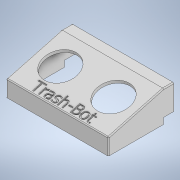
# Autodesk Inventor part: Ultrasonic_Sensor_Holder
Saved by Autodesk Inventor 2020 (Build 240168000, 168)
## iProperties
Created: 2023-02-02
Part Number: Ultrasonic_Sensor_Holder
Material: Generic
Document SubType Name: Modeling
Designer: Matthew Ng
Density: 1 g/cm^3
Appearance: Default
Author: Matthew Ng
Autodesk Inventor part; units mm, degrees
ref_plane "YZ Plane" through (0, 0, 0) normal (1, 0, 0) x (0, 1, 0)
ref_plane "XZ Plane" through (0, 0, 0) normal (0, 1, 0) x (-1, 0, 0)
ref_plane "XY Plane" through (0, 0, 0) normal (0, 0, 1) x (1, 0, 0)
sketch "Sketch1" plane through (0, 0, 0) normal (1, 0, 0) x (0, 1, 0)
  line L0 (0, 0) -> (8, 0)
  line L1 (15.2346, -27) -> (8, 0)
  line L2 (15.2346, -27) -> (15.2346, -32)
  line L3 (15.2346, -32) -> (0, -32)
  line L4 (0, -32) -> (0, 0)
  dimension "d8" = 8
  dimension "d26" = 5
  dimension "d27" = 32
  dimension "d28" = 15.2346
  dimension "d29" = 75
  constraints: 10 end point, 1 horizontal, 1 vertical
  measures "d8" distance of L0.start L0.end
  measures "d26" distance of L2.start L2.end
  measures "d27" distance of L3.end L0.start
  measures "d28" distance of L2.end L3.end
  measures "d29" angle of L3 L1
extrude "Extrusion1" add sketch "Sketch1" against normal blind 50
shell "Shell2" thickness 1.5 removed faces 2 at (-33.3333, 0, -10.6667) at (-33.3333, 5.0782, -32)
sketch "Sketch6" plane through (-50, 15.2346, -27) normal (0, 0.9659258, 0.258819) x (1, 0, 0)
  line L0 (25, -27.9525) -> (25, 4.8296) construction
  point P0 (50, -30.023)
  point P1 (12, -12.9525)
  point P2 (38, -12.9525)
  point P3 (12, -12.9525)
  dimension "d31" = 25.9999
  constraints: 2 end point, 1 coincident, 1 symmetric about line
  measures "d31" distance of point (38, -12.952) point (12, -12.952)
hole "Hole2" at (-38, 11.8823, -14.4889) at (-12, 11.8823, -14.4889) direction (0, -0.9659258, -0.258819) diameter 16 end through all
sketch "Sketch7" plane through (-50, 15.2346, -27) normal (0, 0.9659258, 0.258819) x (1, 0, 0)
  line L0 (12.3611, -21.6967) -> (37.6389, -21.6967) construction
  line L1 (37.6389, -21.6967) -> (37.6389, -26.9518) construction
  line L2 (37.6389, -26.9518) -> (12.3611, -26.9518) construction
  line L3 (12.3611, -26.9518) -> (12.3611, -21.6967) construction
  line L4 (11.8801, -26.9196) -> (11.8801, -22.5111)
  line L5 (11.8801, -22.5111) -> (10.2026, -22.5111)
  line L6 (10.2026, -22.5111) -> (10.2026, -21.9196)
  line L7 (10.2026, -21.9196) -> (14.222, -21.9196)
  line L8 (14.222, -21.9196) -> (14.222, -22.5111)
  line L9 (14.222, -22.5111) -> (12.5446, -22.5111)
  line L10 (12.5446, -22.5111) -> (12.5446, -26.9196)
  line L11 (12.5446, -26.9196) -> (11.8801, -26.9196)
  line L12 (16.6694, -23.8442) -> (16.637, -23.8442)
  spline S0 degree 2 poles (16.637, -23.8442) (16.564, -23.8239) (16.406, -23.8158) (16.2966, -23.8158) knots 0 0 0 1 2 2 2
  spline S1 degree 2 poles (16.2966, -23.8158) (16.0413, -23.8158) (15.5389, -24.0387) (15.312, -24.2575) knots 0 0 0 1 2 2 2
  line L13 (15.312, -24.2575) -> (15.312, -26.9196)
  line L14 (15.312, -26.9196) -> (14.6799, -26.9196)
  line L15 (14.6799, -26.9196) -> (14.6799, -23.1675)
  line L16 (14.6799, -23.1675) -> (15.312, -23.1675)
  line L17 (15.312, -23.1675) -> (15.312, -23.7267)
  spline S2 degree 2 poles (15.312, -23.7267) (15.6564, -23.4188) (16.171, -23.1675) (16.4141, -23.1675) knots 0 0 0 1 2 2 2
  spline S3 degree 2 poles (16.4141, -23.1675) (16.5113, -23.1675) (16.6086, -23.1756) (16.6694, -23.1878) knots 0 0 0 1 2 2 2
  line L18 (16.6694, -23.1878) -> (16.6694, -23.8442)
  spline S4 degree 2 poles (19.2504, -26.5225) (19.1734, -26.5792) (18.9141, -26.7818) (18.7925, -26.8426) knots 0 0 0 1 2 2 2
  spline S5 degree 2 poles (18.7925, -26.8426) (18.6264, -26.9317) (18.3144, -27.0249) (18.0308, -27.0249) knots 0 0 0 1 2 2 2
  spline S6 degree 2 poles (18.0308, -27.0249) (17.7998, -27.0249) (17.3825, -26.8507) (17.2245, -26.6927) knots 0 0 0 1 2 2 2
  spline S7 degree 2 poles (17.2245, -26.6927) (17.0746, -26.5387) (16.8922, -26.0849) (16.8922, -25.8337) knots 0 0 0 1 2 2 2
  spline S8 degree 2 poles (16.8922, -25.8337) (16.8922, -25.4447) (17.2204, -24.8936) (17.577, -24.7356) knots 0 0 0 1 2 2 2
  spline S9 degree 2 poles (17.577, -24.7356) (17.893, -24.5897) (18.752, -24.4803) (19.2504, -24.452) knots 0 0 0 1 2 2 2
  line L19 (19.2504, -24.452) -> (19.2504, -24.3304)
  spline S10 degree 2 poles (19.2504, -24.3304) (19.2504, -24.1116) (19.1167, -23.8402) (18.9951, -23.7632) knots 0 0 0 1 2 2 2
  spline S11 degree 2 poles (18.9951, -23.7632) (18.8736, -23.6862) (18.5251, -23.6376) (18.3387, -23.6376) knots 0 0 0 1 2 2 2
  spline S12 degree 2 poles (18.3387, -23.6376) (18.1199, -23.6376) (17.5284, -23.7672) (17.2326, -23.8928) knots 0 0 0 1 2 2 2
  line L20 (17.2326, -23.8928) -> (17.1961, -23.8928)
  line L21 (17.1961, -23.8928) -> (17.1961, -23.2486)
  spline S13 degree 2 poles (17.1961, -23.2486) (17.3703, -23.2) (18.0227, -23.0784) (18.3428, -23.0784) knots 0 0 0 1 2 2 2
  spline S14 degree 2 poles (18.3428, -23.0784) (18.7318, -23.0784) (19.2626, -23.2) (19.4733, -23.358) knots 0 0 0 1 2 2 2
  spline S15 degree 2 poles (19.4733, -23.358) (19.6799, -23.512) (19.8825, -24.0022) (19.8825, -24.3547) knots 0 0 0 1 2 2 2
  line L22 (19.8825, -24.3547) -> (19.8825, -26.9196)
  line L23 (19.8825, -26.9196) -> (19.2504, -26.9196)
  line L24 (19.2504, -26.9196) -> (19.2504, -26.5225)
  line L25 (19.2504, -25.9957) -> (19.2504, -24.9544)
  spline S16 degree 2 poles (19.2504, -24.9544) (19.0235, -24.9747) (18.3387, -25.0436) (18.124, -25.1084) knots 0 0 0 1 2 2 2
  spline S17 degree 2 poles (18.124, -25.1084) (17.8728, -25.1854) (17.5446, -25.5055) (17.5446, -25.7891) knots 0 0 0 1 2 2 2
  spline S18 degree 2 poles (17.5446, -25.7891) (17.5446, -26.1132) (17.9092, -26.4414) (18.2577, -26.4414) knots 0 0 0 1 2 2 2
  spline S19 degree 2 poles (18.2577, -26.4414) (18.5535, -26.4414) (19.0397, -26.1862) (19.2504, -25.9957) knots 0 0 0 1 2 2 2
  spline S20 degree 2 poles (21.7828, -27.0087) (21.406, -27.0087) (20.7536, -26.8061) (20.5389, -26.6927) knots 0 0 0 1 2 2 2
  line L26 (20.5389, -26.6927) -> (20.5389, -25.9836)
  line L27 (20.5389, -25.9836) -> (20.5713, -25.9836)
  spline S21 degree 2 poles (20.5713, -25.9836) (20.6524, -26.0484) (20.8712, -26.2024) (21.0535, -26.2875) knots 0 0 0 1 2 2 2
  spline S22 degree 2 poles (21.0535, -26.2875) (21.2115, -26.3645) (21.6005, -26.4779) (21.8071, -26.4779) knots 0 0 0 1 2 2 2
  spline S23 degree 2 poles (21.8071, -26.4779) (21.9571, -26.4779) (22.3015, -26.409) (22.3825, -26.3523) knots 0 0 0 1 2 2 2
  spline S24 degree 2 poles (22.3825, -26.3523) (22.5, -26.2753) (22.6053, -26.1011) (22.6053, -25.9228) knots 0 0 0 1 2 2 2
  spline S25 degree 2 poles (22.6053, -25.9228) (22.6053, -25.7) (22.3622, -25.469) (22.0502, -25.392) knots 0 0 0 1 2 2 2
  spline S26 degree 2 poles (22.0502, -25.392) (21.9287, -25.3637) (21.5397, -25.2826) (21.3736, -25.238) knots 0 0 0 1 2 2 2
  spline S27 degree 2 poles (21.3736, -25.238) (20.9441, -25.1124) (20.5551, -24.5938) (20.5551, -24.2251) knots 0 0 0 1 2 2 2
  spline S28 degree 2 poles (20.5551, -24.2251) (20.5551, -23.7145) (21.3209, -23.0784) (21.953, -23.0784) knots 0 0 0 1 2 2 2
  spline S29 degree 2 poles (21.953, -23.0784) (22.265, -23.0784) (22.8971, -23.2324) (23.1118, -23.3499) knots 0 0 0 1 2 2 2
  line L28 (23.1118, -23.3499) -> (23.1118, -24.0265)
  line L29 (23.1118, -24.0265) -> (23.0794, -24.0265)
  spline S30 degree 2 poles (23.0794, -24.0265) (22.8363, -23.832) (22.2447, -23.6092) (21.9408, -23.6092) knots 0 0 0 1 2 2 2
  spline S31 degree 2 poles (21.9408, -23.6092) (21.6288, -23.6092) (21.1994, -23.8726) (21.1994, -24.1359) knots 0 0 0 1 2 2 2
  spline S32 degree 2 poles (21.1994, -24.1359) (21.1994, -24.375) (21.4546, -24.606) (21.7383, -24.6789) knots 0 0 0 1 2 2 2
  spline S33 degree 2 poles (21.7383, -24.6789) (21.876, -24.7154) (22.2245, -24.7883) (22.4149, -24.8329) knots 0 0 0 1 2 2 2
  spline S34 degree 2 poles (22.4149, -24.8329) (22.8282, -24.9382) (23.2496, -25.4204) (23.2496, -25.8377) knots 0 0 0 1 2 2 2
  spline S35 degree 2 poles (23.2496, -25.8377) (23.2496, -26.0808) (23.0592, -26.5103) (22.8728, -26.6684) knots 0 0 0 1 2 2 2
  spline S36 degree 2 poles (22.8728, -26.6684) (22.6742, -26.8345) (22.1677, -27.0087) (21.7828, -27.0087) knots 0 0 0 1 2 2 2
  line L30 (26.7828, -26.9196) -> (26.1507, -26.9196)
  line L31 (26.1507, -26.9196) -> (26.1507, -24.7802)
  spline S37 degree 2 poles (26.1507, -24.7802) (26.1507, -24.5209) (26.1021, -24.0752) (26.0292, -23.9414) knots 0 0 0 1 2 2 2
  spline S38 degree 2 poles (26.0292, -23.9414) (25.9522, -23.7996) (25.6767, -23.6619) (25.4417, -23.6619) knots 0 0 0 1 2 2 2
  spline S39 degree 2 poles (25.4417, -23.6619) (25.2066, -23.6619) (24.7083, -23.9131) (24.4692, -24.1157) knots 0 0 0 1 2 2 2
  line L32 (24.4692, -24.1157) -> (24.4692, -26.9196)
  line L33 (24.4692, -26.9196) -> (23.8371, -26.9196)
  line L34 (23.8371, -26.9196) -> (23.8371, -21.6967)
  line L35 (23.8371, -21.6967) -> (24.4692, -21.6967)
  line L36 (24.4692, -21.6967) -> (24.4692, -23.5849)
  spline S40 degree 2 poles (24.4692, -23.5849) (24.7528, -23.3296) (25.2998, -23.0622) (25.6078, -23.0622) knots 0 0 0 1 2 2 2
  spline S41 degree 2 poles (25.6078, -23.0622) (26.1588, -23.0622) (26.7828, -23.7915) (26.7828, -24.4844) knots 0 0 0 1 2 2 2
  line L37 (26.7828, -24.4844) -> (26.7828, -26.9196)
  line L38 (29.4084, -25.0355) -> (27.5162, -25.0355)
  line L39 (27.5162, -25.0355) -> (27.5162, -24.4277)
  line L40 (27.5162, -24.4277) -> (29.4084, -24.4277)
  line L41 (29.4084, -24.4277) -> (29.4084, -25.0355)
  spline S42 degree 2 poles (33.6062, -25.3839) (33.6062, -25.7567) (33.3225, -26.328) (33.0875, -26.5144) knots 0 0 0 1 2 2 2
  spline S43 degree 2 poles (33.0875, -26.5144) (32.8039, -26.7332) (32.1596, -26.9196) (31.6491, -26.9196) knots 0 0 0 1 2 2 2
  line L42 (31.6491, -26.9196) -> (30.2147, -26.9196)
  line L43 (30.2147, -26.9196) -> (30.2147, -21.9196)
  line L44 (30.2147, -21.9196) -> (31.5397, -21.9196)
  spline S44 degree 2 poles (31.5397, -21.9196) (32.0746, -21.9196) (32.6094, -21.9884) (32.8525, -22.1222) knots 0 0 0 1 2 2 2
  spline S45 degree 2 poles (32.8525, -22.1222) (33.124, -22.264) (33.3712, -22.7299) (33.3712, -23.046) knots 0 0 0 1 2 2 2
  spline S46 degree 2 poles (33.3712, -23.046) (33.3712, -23.3985) (32.9984, -23.9577) (32.6702, -24.1157) knots 0 0 0 1 2 2 2
  line L45 (32.6702, -24.1157) -> (32.6702, -24.14)
  spline S47 degree 2 poles (32.6702, -24.14) (33.1159, -24.2615) (33.6062, -24.9058) (33.6062, -25.3839) knots 0 0 0 1 2 2 2
  spline S48 degree 2 poles (32.9133, -25.4123) (32.9133, -25.1286) (32.7512, -24.764) (32.5081, -24.6343) knots 0 0 0 1 2 2 2
  spline S49 degree 2 poles (32.5081, -24.6343) (32.3501, -24.5533) (31.9773, -24.5047) (31.6329, -24.5047) knots 0 0 0 1 2 2 2
  line L46 (31.6329, -24.5047) -> (30.8793, -24.5047)
  line L47 (30.8793, -24.5047) -> (30.8793, -26.3523)
  line L48 (30.8793, -26.3523) -> (31.4182, -26.3523)
  spline S50 degree 2 poles (31.4182, -26.3523) (31.8558, -26.3523) (32.3582, -26.2713) (32.5527, -26.1416) knots 0 0 0 1 2 2 2
  spline S51 degree 2 poles (32.5527, -26.1416) (32.7391, -26.0079) (32.9133, -25.6756) (32.9133, -25.4123) knots 0 0 0 1 2 2 2
  spline S52 degree 2 poles (32.6783, -23.1392) (32.6783, -22.9609) (32.5567, -22.6935) (32.423, -22.6165) knots 0 0 0 1 2 2 2
  spline S53 degree 2 poles (32.423, -22.6165) (32.2609, -22.5273) (31.8679, -22.4868) (31.5154, -22.4868) knots 0 0 0 1 2 2 2
  line L49 (31.5154, -22.4868) -> (30.8793, -22.4868)
  line L50 (30.8793, -22.4868) -> (30.8793, -23.9496)
  line L51 (30.8793, -23.9496) -> (31.6329, -23.9496)
  spline S54 degree 2 poles (31.6329, -23.9496) (31.9449, -23.9496) (32.2407, -23.8847) (32.3987, -23.7834) knots 0 0 0 1 2 2 2
  spline S55 degree 2 poles (32.3987, -23.7834) (32.5527, -23.6862) (32.6783, -23.3742) (32.6783, -23.1392) knots 0 0 0 1 2 2 2
  spline S56 degree 2 poles (37.3015, -25.0436) (37.3015, -25.9917) (36.3898, -27.0249) (35.628, -27.0249) knots 0 0 0 1 2 2 2
  spline S57 degree 2 poles (35.628, -27.0249) (34.846, -27.0249) (33.9506, -25.9593) (33.9506, -25.0436) knots 0 0 0 1 2 2 2
  spline S58 degree 2 poles (33.9506, -25.0436) (33.9506, -24.1035) (34.8744, -23.0622) (35.628, -23.0622) knots 0 0 0 1 2 2 2
  spline S59 degree 2 poles (35.628, -23.0622) (36.3898, -23.0622) (37.3015, -24.0995) (37.3015, -25.0436) knots 0 0 0 1 2 2 2
  spline S60 degree 2 poles (36.6491, -25.0436) (36.6491, -24.3142) (36.1183, -23.6051) (35.628, -23.6051) knots 0 0 0 1 2 2 2
  spline S61 degree 2 poles (35.628, -23.6051) (35.1378, -23.6051) (34.6029, -24.3142) (34.6029, -25.0436) knots 0 0 0 1 2 2 2
  spline S62 degree 2 poles (34.6029, -25.0436) (34.6029, -25.7526) (35.1378, -26.482) (35.628, -26.482) knots 0 0 0 1 2 2 2
  spline S63 degree 2 poles (35.628, -26.482) (36.1143, -26.482) (36.6491, -25.7648) (36.6491, -25.0436) knots 0 0 0 1 2 2 2
  spline S64 degree 2 poles (39.0843, -26.9925) (38.5697, -26.9925) (37.9903, -26.405) (37.9903, -25.7688) knots 0 0 0 1 2 2 2
  line L52 (37.9903, -25.7688) -> (37.9903, -23.6902)
  line L53 (37.9903, -23.6902) -> (37.5648, -23.6902)
  line L54 (37.5648, -23.6902) -> (37.5648, -23.1675)
  line L55 (37.5648, -23.1675) -> (37.9903, -23.1675)
  line L56 (37.9903, -23.1675) -> (37.9903, -22.0897)
  line L57 (37.9903, -22.0897) -> (38.6224, -22.0897)
  line L58 (38.6224, -22.0897) -> (38.6224, -23.1675)
  line L59 (38.6224, -23.1675) -> (39.7853, -23.1675)
  line L60 (39.7853, -23.1675) -> (39.7853, -23.6902)
  line L61 (39.7853, -23.6902) -> (38.6224, -23.6902)
  line L62 (38.6224, -23.6902) -> (38.6224, -25.4771)
  spline S65 degree 2 poles (38.6224, -25.4771) (38.6224, -25.7607) (38.6426, -26.0727) (38.7115, -26.2064) knots 0 0 0 1 2 2 2
  spline S66 degree 2 poles (38.7115, -26.2064) (38.7682, -26.3239) (39.0235, -26.4414) (39.2423, -26.4414) knots 0 0 0 1 2 2 2
  spline S67 degree 2 poles (39.2423, -26.4414) (39.3963, -26.4414) (39.684, -26.3483) (39.7488, -26.3199) knots 0 0 0 1 2 2 2
  line L63 (39.7488, -26.3199) -> (39.7853, -26.3199)
  line L64 (39.7853, -26.3199) -> (39.7853, -26.8872)
  spline S68 degree 2 poles (39.7853, -26.8872) (39.607, -26.9358) (39.2423, -26.9925) (39.0843, -26.9925) knots 0 0 0 1 2 2 2
  point P0 (50, -30.023)
  constraints: 2 other
emboss "Emboss1" sketch "Sketch7" operation cut depth 0.5 direction (0, -0.9659258, -0.258819)
fillet "Fillet1" radius 0.5 7 edges at (-25, 8, 0) (0, 11.6173, -13.5) (0, 4, 0) (-50, 4, 0) (-50, 11.6173, -13.5) (-50, 15.2346, -29.5) (0, 15.2346, -29.5)
sketch "Sketch8" plane through (0, 0, 0) normal (1, 0, 0) x (0, 0, -1)
  line L0 (0.5, 0) -> (32, 0) projected
  line L1 (32, 0) -> (27, 0)
  line L2 (27, 0) -> (27, 3)
  line L3 (27, 3) -> (32, 3)
  line L4 (32, 3) -> (32, 0)
  point P0 (0, 0)
  dimension "d43" = 5
  dimension "d44" = 3
  constraints: 8 end point, 2 parallel, 1 horizontal, 1 perpendicular
  measures "d43" distance of L2.end L3.end
  measures "d44" distance of L1.end L2.end
extrude "Extrusion3" cut sketch "Sketch8" against normal blind 50
body "Solid1"
